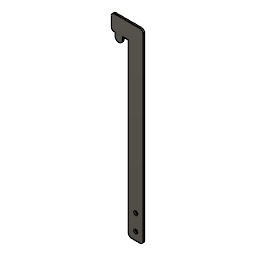
_Shelf Hangermount2.d744eca5-0801-4c6a-ae0e-8c6e70867a54 (Autodesk Fusion 360 design; units mm, degrees)
Autodesk Fusion 360 part; units mm, degrees
sketch "Sketch1" plane through (0, 0, 0) normal (0, 0, 1) x (1, 0, 0)
  line L0 (50.8, 180.4) -> (50.8, -60)
  circle A0 centre (38.9, -72.7) radius 3
  line L1 (18, 160) -> (18, 155)
  line L2 (50.8, -110.8) -> (27, -85.4) construction
  arc A1 (6, 155) -> (18, 155) centre (12, 155) ccw
  line L3 (50.8, -60) -> (50.8, -105.8)
  arc A2 (50.8, 180.4) -> (45.8, 185.4) centre (45.8, 180.4) ccw
  line L4 (18, 160) -> (27, 160)
  arc A3 (27, -105.8) -> (32, -110.8) centre (32, -105.8) ccw
  arc A4 (5, 185.4) -> (0, 180.4) centre (5, 180.4) ccw
  circle A5 centre (38.9, -98.1) radius 3
  line L5 (5, 185.4) -> (45.8, 185.4)
  line L6 (12, 160) -> (12, 155) construction
  line L7 (27, 160) -> (27, -60)
  line L8 (27, -60) -> (50.8, -60) construction
  line L9 (6, 160) -> (6, 155)
  line L10 (5, 160) -> (6, 160)
  line L11 (0, 165) -> (0, 180.4)
  arc A6 (45.8, -110.8) -> (50.8, -105.8) centre (45.8, -105.8) ccw
  arc A7 (0, 165) -> (5, 160) centre (5, 165) ccw
  line L12 (6, 160) -> (18, 160) construction
  line L13 (27, -105.8) -> (27, -60)
  line L14 (45.8, -110.8) -> (32, -110.8)
  line L15 (50.8, -60) -> (27, -85.4) construction
  point P0 (0, 160)
  point P1 (0, 185.4)
  point P2 (50.8, 185.4)
  point P3 (0, 160)
  point P4 (27, -110.8)
  dimension "d1" = 50.8
  dimension "d2" = 25.4
  dimension "d3" = 6
  dimension "d4" = 5
  dimension "d5" = 220
  dimension "d6" = 50.8
  dimension "d7" = 6
  dimension "d8" = 6
  dimension "d9" = 5
  constraint coincident P3 P0
  constraint vertical L11
  constraint perpendicular L5 L11
  constraint perpendicular L10 L11
  constraint parallel L10 L12
  constraint midpoint L6.start L12
  constraint perpendicular L6 L12
  constraint coincident A1.centre L6.end
  constraint tangent A1 L9
  constraint perpendicular L9 L12
  constraint tangent L1 A1
  constraint perpendicular L1 L4
  constraint perpendicular L4 L7
  constraint perpendicular L0 L5
  constraint horizontal L8
  constraint vertical L3
  constraint horizontal L14
  constraint vertical L13
  constraint midpoint A0.centre L15
  constraint midpoint A5.centre L2
  constraint equal A0 A5
  constraint coincident P1 L11
  constraint coincident P1 L5
  constraint tangent A4 L11
  constraint tangent A4 L5
  constraint coincident P2 L5
  constraint coincident P2 L0
  constraint tangent A2 L5
  constraint tangent L0 A2
  constraint equal A2 A4
  constraint coincident L2.start L14
  constraint coincident L2.start L3
  constraint tangent A6 L14
  constraint tangent L3 A6
  constraint equal A4 A6
  constraint coincident L2.end L13
  constraint coincident P4 L13
  constraint coincident P4 L14
  constraint tangent A3 L13
  constraint tangent A3 L14
  constraint equal A3 A4
  constraint coincident P3 L10
  constraint coincident P3 L11
  constraint tangent L10 A7
  constraint tangent L11 A7
  constraint equal A4 A7
  measures "d1" distance of P1 P2
  measures "d2" distance of P3 P1
  measures "d3" distance of P3 L9.start
  measures "d4" distance of L6.start A1.centre
  measures "d5" distance of L4.end L7.end
  measures "d6" distance of L7.end P4
  measures "d7" diameter of A0
  measures "d8" radius of A1
  measures "d9" radius of A4
extrude "BaseFlange1" add sketch "Sketch1" along normal blind 2.5
